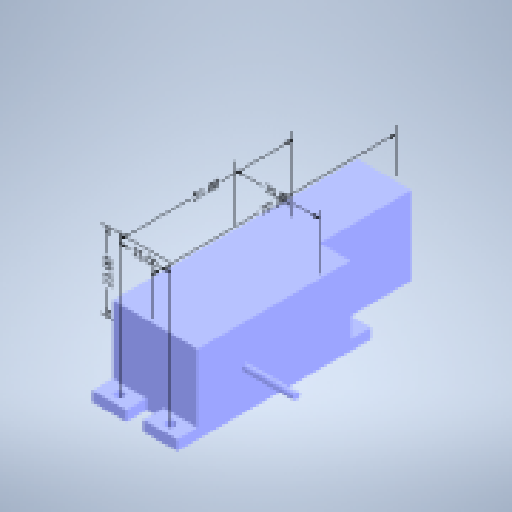
# Autodesk Inventor part: motor
Saved by Autodesk Inventor 2024.1 (Build 281209000, 209)
## iProperties
Created: 2024-11-09
Part Number: motor
Material: ガラス
Document SubType Name: Modeling
Designer: hibik
Density: 2.18 g/cm^3
Appearance: クリア
Author: hibik
Autodesk Inventor part; units mm, degrees
ref_plane "YZ Plane" through (0, 0, 0) normal (1, 0, 0) x (0, 1, 0)
ref_plane "XZ Plane" through (0, 0, 0) normal (0, 1, 0) x (-1, 0, 0)
ref_plane "XY Plane" through (0, 0, 0) normal (0, 0, 1) x (1, 0, 0)
sketch "スケッチ1" plane through (0, 0, 0) normal (0, 1, 0) x (-1, 0, 0)
  line L0 (0, 0) -> (25, 0)
  line L1 (25, 0) -> (25, -45)
  line L2 (25, -45) -> (0, -45)
  line L3 (0, -45) -> (0, 0)
  line L4 (9, -45) -> (25, -45)
  line L5 (25, -45) -> (25, -72)
  line L6 (25, -72) -> (9, -72)
  line L7 (9, -72) -> (9, -45)
  point P0 (25, -45)
  dimension "d0" = 25
  dimension "d1" = 45
  dimension "d2" = 16
  dimension "d3" = 27
  constraints: 16 end point, 4 parallel, 2 collinear, 2 horizontal, 2 perpendicular
  measures "d0" distance of L2.end L1.end
  measures "d1" distance of L0.end L1.end
  measures "d2" distance of L5.end L6.end
  measures "d3" distance of L4.end L5.end
extrude "押し出し1" add sketch "スケッチ1" along normal blind 23
sketch "スケッチ2" plane through (-25, 0, -45) normal (-1, 0, 0) x (0, 0, 1)
  circle A0 centre (31, 11.5) radius 1
  line L0 (45, 0) -> (45, 23) projected
  point P0 (45, 11.5)
  dimension "d6" = 2
  dimension "d7" = 14
  constraints: 1 centre point, 1 horizontal alignment, 1 midpoint
  measures "d6" diameter of A0
  measures "d7" distance from line of L0 A0.centre
extrude "押し出し2" add sketch "スケッチ2" against normal blind 40
sketch "スケッチ3" plane through (0, 0, 0) normal (0, -1, 0) x (1, 0, 0)
  circle A0 centre (-20, 3) radius 1.35
  circle A1 centre (-5, 3) radius 1.35
  line L0 (-25, -72) -> (-25, 0) projected
  line L1 (-25, 0) -> (0, 0) projected
  line L2 (-25, 0) -> (-15, 0)
  line L3 (-15, 0) -> (-15, 6)
  line L4 (-15, 6) -> (-25, 6)
  line L5 (-25, 6) -> (-25, 0)
  line L6 (0, 0) -> (-10, 0)
  line L7 (-10, 0) -> (-10, 6)
  line L8 (-10, 6) -> (0, 6)
  line L9 (0, 6) -> (0, 0)
  circle A2 centre (-5, -48) radius 1.35
  line L10 (-25, -72) -> (-25, -45) projected
  line L11 (-25, -45) -> (-25, -45)
  line L12 (-25, -45) -> (-25, -51)
  line L13 (-25, -51) -> (-25, -51)
  line L14 (-25, -51) -> (-25, -45)
  line L15 (-9, -45) -> (-9, -72) projected
  line L16 (-9, -45) -> (0, -45)
  line L17 (0, -45) -> (0, -51)
  line L18 (0, -51) -> (-9, -51)
  line L19 (-9, -51) -> (-9, -45)
  line L20 (0, 0) -> (0, -45) projected
  point P0 (-16, -45)
  point P1 (-16, -45)
  point P2 (-5, 6)
  dimension "d10" = 2.7
  dimension "d11" = 2.7
  dimension "d12" = 5
  dimension "d14" = 3
  dimension "d15" = 3
  dimension "d16" = 10
  dimension "d17" = 6
  dimension "d20" = 2.7
  dimension "d21" = 3
  dimension "d22" = 6
  dimension "d34" = 6
  constraints: 32 end point, 8 equal length, 4 horizontal, 4 perpendicular, 3 centre point, 2 collinear, 2 vertical alignment, 1 midpoint, 1 point on line, 2 other
  measures "d10" diameter of A0
  measures "d11" diameter of A1
  measures "d12" distance from line of L0 A0.centre
  measures "d14" distance from line of L1 A0.centre
  measures "d15" distance from line of L1 A1.centre
  measures "d16" distance of L3.end L4.end
  measures "d17" distance of L4.end L0.end
  measures "d20" diameter of A2
  measures "d21" distance from line of L11 A2.centre
  measures "d22" distance of L13.end L11.start
  measures "d34" distance of L16.end L17.end
extrude "押し出し3" add sketch "スケッチ3" against normal blind 3
equation "\"d15\" = d14"
equation "\"d16\" = 2 * d12"
equation "\"d34\" = d17"
